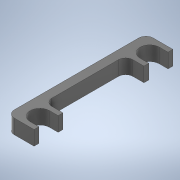
# Autodesk Inventor part: Base
Saved by Autodesk Inventor 2020.2 (Build 242310000, 310)
## iProperties
Created: 2021-06-22
Part Number: Base
Material: Generic
Document SubType Name: Modeling
Designer: JK
Density: 1 g/cm^3
Appearance: Smooth - Black
Author: JK
Autodesk Inventor part; units mm, degrees
ref_plane "YZ Plane" through (0, 0, 0) normal (1, 0, 0) x (0, 1, 0)
ref_plane "XZ Plane" through (0, 0, 0) normal (0, 1, 0) x (-1, 0, 0)
ref_plane "XY Plane" through (0, 0, 0) normal (0, 0, 1) x (1, 0, 0)
sketch "Sketch1" plane through (0, 0, 0) normal (0, 1, 0) x (-1, 0, 0)
  circle A0 centre (0, 38) radius 6.65
  circle A1 centre (0, -38) radius 6.65
  circle A2 centre (0, 38) radius 10
  circle A3 centre (0, -38) radius 10
  line L0 (6.65, 48) -> (12.65, 48)
  line L1 (12.65, 48) -> (12.65, -48)
  line L2 (12.65, -48) -> (6.65, -48)
  line L3 (6.65, -48) -> (6.65, 48)
  line L4 (12.65, 48) -> (0, 48)
  line L5 (12.65, -48) -> (0, -48)
  line L6 (0, 28) -> (6.65, 28)
  line L7 (0, -28) -> (6.65, -28)
  line L8 (0, 48) -> (0, -48)
  point P0 (0, 0)
  point P1 (0, 31.35)
  point P2 (0, -31.35)
  point P3 (0, -44.65)
  point P4 (6.65, -45.4684)
  point P5 (0, 44.65)
  dimension "d0" = 38
  dimension "d1" = 38
  dimension "d2" = 13.3
  dimension "d3" = 20
  dimension "d4" = 20
  dimension "d5" = 6
  constraints: 18 end point, 4 centre point, 4 point on circle, 3 perpendicular, 3 point on line, 3 tangent, 2 coincident, 2 parallel, 1 equal radius, 1 horizontal, 1 vertical
  measures "d0" distance of point (0, 0) A0.centre
  measures "d1" distance of point (0, 0) A1.centre
  measures "d2" diameter of A0
  measures "d3" diameter of A2
  measures "d4" diameter of A3
  measures "d5" distance between parallel lines of L1 L3
extrude "Extrusion1" add sketch "Sketch1" along normal blind 10 contours L3 A2 L8 A0 | L3 A2 | A0 L8 A2 L3 | L3 L6 A2 | A2 L3 L0 L1 L2 A3 | A2 L4 L3 | L7 L3 A3 | A3 L3 A1 L8 | L8 A1 L3 A3 | A3 L3 L5 | A3 L3
fillet "Fillet1" radius 5 4 edges at (-12.65, 5, 48) (-12.65, 5, -48) (-6.65, 5, -28) (-6.65, 5, 28)
sketch "Sketch2" plane through (0, 0, -44.65) normal (1, 0, 0) x (0, 0, -1)
  line L0 (0, 0) -> (3.35, 0) projected
  line L1 (3.35, 0) -> (3.35, 10) projected
  line L2 (0, 10) -> (3.35, 10) projected
  line L3 (0, 0) -> (0, 10) projected
  line L4 (-16.65, 0) -> (-13.3, 0) projected
  line L5 (-13.3, 0) -> (-13.3, 10) projected
  line L6 (-16.65, 10) -> (-13.3, 10) projected
  line L7 (-16.65, 0) -> (-16.65, 10) projected
  line L8 (-76, 0) -> (-72.65, 0) projected
  line L9 (-72.65, 0) -> (-72.65, 10) projected
  line L10 (-76, 10) -> (-72.65, 10) projected
  line L11 (-76, 0) -> (-76, 10) projected
  line L12 (-92.65, 0) -> (-89.3, 0) projected
  line L13 (-89.3, 0) -> (-89.3, 10) projected
  line L14 (-92.65, 10) -> (-89.3, 10) projected
  line L15 (-92.65, 0) -> (-92.65, 10) projected
  point P0 (-44.65, 0)
extrude "Extrusion2" add sketch "Sketch2" along normal blind 6
body "Solid1"
